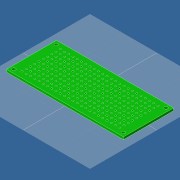
# Autodesk Inventor part: PCB_70x30
Saved by Autodesk Inventor 2016 SP2 (Build 200236200, 236)
## iProperties
Created: 2017-11-11
Part Number: PCB_70x30
Material: Generisch
Document SubType Name: Modeling
Designer: User
Density: 1 g/cm^3
Appearance: Dunkelgrün
Author: User
Autodesk Inventor part; units mm, degrees
ref_plane "YZ Plane" through (0, 0, 0) normal (1, 0, 0) x (0, 1, 0)
ref_plane "XZ Plane" through (0, 0, 0) normal (0, 1, 0) x (-1, 0, 0)
ref_plane "XY Plane" through (0, 0, 0) normal (0, 0, 1) x (1, 0, 0)
sketch "Skizze1" plane through (0, 0, 0) normal (0, 0, 1) x (1, 0, 0)
  line L0 (35, -15) -> (-35, -15)
  line L1 (-35, -15) -> (-35, 15)
  line L2 (-35, 15) -> (35, 15)
  line L3 (35, 15) -> (35, -15)
  line L4 (35, -15) -> (-35, 15) construction
  line L5 (-35, -15) -> (35, 15) construction
  circle A0 centre (-32.75, 12.75) radius 1
  circle A1 centre (-32.75, -12.75) radius 1
  circle A2 centre (32.75, 12.75) radius 1
  circle A3 centre (32.75, -12.75) radius 1
  line L6 (-49, 0) -> (49, 0) construction
  line L7 (0, -21) -> (0, 21) construction
  point P0 (0, 0)
  dimension "d0" = 70
  dimension "d1" = 30
  dimension "d45" = 2
  dimension "d46" = 65.5
  dimension "d47" = 25.5
  constraints: 12 end point, 4 centre point, 3 equal radius, 2 horizontal alignment, 2 midpoint, 2 parallel, 2 symmetric about line, 2 vertical alignment, 1 horizontal, 1 perpendicular
  measures "d0" distance of L1.end L2.end
  measures "d1" distance of L0.end L1.end
  measures "d45" diameter of A0
  measures "d46" distance of A2.centre A0.centre
  measures "d47" distance of A3.centre A2.centre
extrude "Extrusion1" add sketch "Skizze1" along normal blind 1.5 contours L0 L1 L2 L3 | A0 | A1 | A2 | A3
sketch "Skizze2" plane through (0, 0, 1.5) normal (0, 0, 1) x (1, 0, 0)
  line L0 (-49, 0) -> (49, 0) projected
  line L1 (0, -23.114) -> (0, 23.114) projected
  point P0 (0, 0)
  point P1 (-1.27, 1.27)
  point P2 (1.27, 1.27)
  point P3 (1.27, -1.27)
  point P4 (-1.27, -1.27)
  point P5 (-1.27, 3.81)
  point P6 (-1.27, 6.35)
  point P7 (-1.27, 8.89)
  point P8 (-1.27, 11.43)
  point P9 (-3.81, 1.27)
  point P10 (-3.81, 3.81)
  point P11 (-3.81, 6.35)
  point P12 (-3.81, 8.89)
  point P13 (-3.81, 11.43)
  point P14 (-6.35, 1.27)
  point P15 (-6.35, 3.81)
  point P16 (-6.35, 6.35)
  point P17 (-6.35, 8.89)
  point P18 (-6.35, 11.43)
  point P19 (-8.89, 1.27)
  point P20 (-8.89, 3.81)
  point P21 (-8.89, 6.35)
  point P22 (-8.89, 8.89)
  point P23 (-8.89, 11.43)
  point P24 (-11.43, 1.27)
  point P25 (-11.43, 3.81)
  point P26 (-11.43, 6.35)
  point P27 (-11.43, 8.89)
  point P28 (-11.43, 11.43)
  point P29 (-13.97, 1.27)
  point P30 (-13.97, 3.81)
  point P31 (-13.97, 6.35)
  point P32 (-13.97, 8.89)
  point P33 (-13.97, 11.43)
  point P34 (-16.51, 1.27)
  point P35 (-16.51, 3.81)
  point P36 (-16.51, 6.35)
  point P37 (-16.51, 8.89)
  point P38 (-16.51, 11.43)
  point P39 (-19.05, 1.27)
  point P40 (-19.05, 3.81)
  point P41 (-19.05, 6.35)
  point P42 (-19.05, 8.89)
  point P43 (-19.05, 11.43)
  point P44 (-21.59, 1.27)
  point P45 (-21.59, 3.81)
  point P46 (-21.59, 6.35)
  point P47 (-21.59, 8.89)
  point P48 (-21.59, 11.43)
  point P49 (-24.13, 1.27)
  point P50 (-24.13, 3.81)
  point P51 (-24.13, 6.35)
  point P52 (-24.13, 8.89)
  point P53 (-24.13, 11.43)
  point P54 (3.81, 1.27)
  point P55 (6.35, 1.27)
  point P56 (8.89, 1.27)
  point P57 (11.43, 1.27)
  point P58 (13.97, 1.27)
  point P59 (16.51, 1.27)
  point P60 (19.05, 1.27)
  point P61 (21.59, 1.27)
  point P62 (24.13, 1.27)
  point P63 (1.27, 3.81)
  point P64 (3.81, 3.81)
  point P65 (6.35, 3.81)
  point P66 (8.89, 3.81)
  point P67 (11.43, 3.81)
  point P68 (13.97, 3.81)
  point P69 (16.51, 3.81)
  point P70 (19.05, 3.81)
  point P71 (21.59, 3.81)
  point P72 (24.13, 3.81)
  point P73 (1.27, 6.35)
  point P74 (3.81, 6.35)
  point P75 (6.35, 6.35)
  point P76 (8.89, 6.35)
  point P77 (11.43, 6.35)
  point P78 (13.97, 6.35)
  point P79 (16.51, 6.35)
  point P80 (19.05, 6.35)
  point P81 (21.59, 6.35)
  point P82 (24.13, 6.35)
  point P83 (1.27, 8.89)
  point P84 (3.81, 8.89)
  point P85 (6.35, 8.89)
  point P86 (8.89, 8.89)
  point P87 (11.43, 8.89)
  point P88 (13.97, 8.89)
  point P89 (16.51, 8.89)
  point P90 (19.05, 8.89)
  point P91 (21.59, 8.89)
  point P92 (24.13, 8.89)
  point P93 (1.27, 11.43)
  point P94 (3.81, 11.43)
  point P95 (6.35, 11.43)
  point P96 (8.89, 11.43)
  point P97 (11.43, 11.43)
  point P98 (13.97, 11.43)
  point P99 (16.51, 11.43)
  point P100 (19.05, 11.43)
  point P101 (21.59, 11.43)
  point P102 (24.13, 11.43)
  point P103 (-1.27, -3.81)
  point P104 (-1.27, -6.35)
  point P105 (-1.27, -8.89)
  point P106 (-1.27, -11.43)
  point P107 (-3.81, -1.27)
  point P108 (-3.81, -3.81)
  point P109 (-3.81, -6.35)
  point P110 (-3.81, -8.89)
  point P111 (-3.81, -11.43)
  point P112 (-6.35, -1.27)
  point P113 (-6.35, -3.81)
  point P114 (-6.35, -6.35)
  point P115 (-6.35, -8.89)
  point P116 (-6.35, -11.43)
  point P117 (-8.89, -1.27)
  point P118 (-8.89, -3.81)
  point P119 (-8.89, -6.35)
  point P120 (-8.89, -8.89)
  point P121 (-8.89, -11.43)
  point P122 (-11.43, -1.27)
  point P123 (-11.43, -3.81)
  point P124 (-11.43, -6.35)
  point P125 (-11.43, -8.89)
  point P126 (-11.43, -11.43)
  point P127 (-13.97, -1.27)
  point P128 (-13.97, -3.81)
  point P129 (-13.97, -6.35)
  point P130 (-13.97, -8.89)
  point P131 (-13.97, -11.43)
  point P132 (-16.51, -1.27)
  point P133 (-16.51, -3.81)
  point P134 (-16.51, -6.35)
  point P135 (-16.51, -8.89)
  point P136 (-16.51, -11.43)
  point P137 (-19.05, -1.27)
  point P138 (-19.05, -3.81)
  point P139 (-19.05, -6.35)
  point P140 (-19.05, -8.89)
  point P141 (-19.05, -11.43)
  point P142 (-21.59, -1.27)
  point P143 (-21.59, -3.81)
  point P144 (-21.59, -6.35)
  point P145 (-21.59, -8.89)
  point P146 (-21.59, -11.43)
  point P147 (-24.13, -1.27)
  point P148 (-24.13, -3.81)
  point P149 (-24.13, -6.35)
  point P150 (-24.13, -8.89)
  point P151 (-24.13, -11.43)
  point P152 (1.27, -3.81)
  point P153 (1.27, -6.35)
  point P154 (1.27, -8.89)
  point P155 (1.27, -11.43)
  point P156 (3.81, -1.27)
  point P157 (3.81, -3.81)
  point P158 (3.81, -6.35)
  point P159 (3.81, -8.89)
  point P160 (3.81, -11.43)
  point P161 (6.35, -1.27)
  point P162 (6.35, -3.81)
  point P163 (6.35, -6.35)
  point P164 (6.35, -8.89)
  point P165 (6.35, -11.43)
  point P166 (8.89, -1.27)
  point P167 (8.89, -3.81)
  point P168 (8.89, -6.35)
  point P169 (8.89, -8.89)
  point P170 (8.89, -11.43)
  point P171 (11.43, -1.27)
  point P172 (11.43, -3.81)
  point P173 (11.43, -6.35)
  point P174 (11.43, -8.89)
  point P175 (11.43, -11.43)
  point P176 (13.97, -1.27)
  point P177 (13.97, -3.81)
  point P178 (13.97, -6.35)
  point P179 (13.97, -8.89)
  point P180 (13.97, -11.43)
  point P181 (16.51, -1.27)
  point P182 (16.51, -3.81)
  point P183 (16.51, -6.35)
  point P184 (16.51, -8.89)
  point P185 (16.51, -11.43)
  point P186 (19.05, -1.27)
  point P187 (19.05, -3.81)
  point P188 (19.05, -6.35)
  point P189 (19.05, -8.89)
  point P190 (19.05, -11.43)
  point P191 (21.59, -1.27)
  point P192 (21.59, -3.81)
  point P193 (21.59, -6.35)
  point P194 (21.59, -8.89)
  point P195 (21.59, -11.43)
  point P196 (24.13, -1.27)
  point P197 (24.13, -3.81)
  point P198 (24.13, -6.35)
  point P199 (24.13, -8.89)
  dimension "d4" = 2.54
  dimension "d5" = 2.54
  dimension "d8" = 2.54
  dimension "d11" = 2.54
  dimension "d16" = 2.54
  dimension "d19" = 2.54
  dimension "d24" = 2.54
  dimension "d27" = 2.54
  dimension "d32" = 2.54
  dimension "d35" = 2.54
  constraints: 4 horizontal, 4 vertical, 2 horizontal alignment, 2 symmetric about line, 2 vertical alignment, 236 other
  measures "d4" distance of point (1.27, 1.27) point (-1.27, 1.27)
  measures "d5" distance of point (-1.27, -1.27) point (-1.27, 1.27)
  measures "d8" distance of point (-1.27, 1.27) point (-1.27, 3.81)
  measures "d11" distance of point (-1.27, 1.27) point (-3.81, 1.27)
  measures "d16" distance of point (1.27, 1.27) point (3.81, 1.27)
  measures "d19" distance of point (1.27, 1.27) point (1.27, 3.81)
  measures "d24" distance of point (-1.27, -1.27) point (-1.27, -3.81)
  measures "d27" distance of point (-1.27, -1.27) point (-3.81, -1.27)
  measures "d32" distance of point (1.27, -1.27) point (1.27, -3.81)
  measures "d35" distance of point (1.27, -1.27) point (3.81, -1.27)
hole "Bohrung1" at (-1.27, 1.27, 1.5) at (1.27, 1.27, 1.5) at (1.27, -1.27, 1.5) at (-1.27, -1.27, 1.5) at (-1.27, 3.81, 1.5) at (-1.27, 6.35, 1.5) at (-1.27, 8.89, 1.5) at (-1.27, 11.43, 1.5) at (-3.81, 1.27, 1.5) at (-3.81, 3.81, 1.5) at (-3.81, 6.35, 1.5) at (-3.81, 8.89, 1.5) at (-3.81, 11.43, 1.5) at (-6.35, 1.27, 1.5) at (-6.35, 3.81, 1.5) at (-6.35, 6.35, 1.5) at (-6.35, 8.89, 1.5) at (-6.35, 11.43, 1.5) at (-8.89, 1.27, 1.5) at (-8.89, 3.81, 1.5) at (-8.89, 6.35, 1.5) at (-8.89, 8.89, 1.5) at (-8.89, 11.43, 1.5) at (-11.43, 1.27, 1.5) at (-11.43, 3.81, 1.5) at (-11.43, 6.35, 1.5) at (-11.43, 8.89, 1.5) at (-11.43, 11.43, 1.5) at (-13.97, 1.27, 1.5) at (-13.97, 3.81, 1.5) at (-13.97, 6.35, 1.5) at (-13.97, 8.89, 1.5) at (-13.97, 11.43, 1.5) at (-16.51, 1.27, 1.5) at (-16.51, 3.81, 1.5) at (-16.51, 6.35, 1.5) at (-16.51, 8.89, 1.5) at (-16.51, 11.43, 1.5) at (-19.05, 1.27, 1.5) at (-19.05, 3.81, 1.5) at (-19.05, 6.35, 1.5) at (-19.05, 8.89, 1.5) at (-19.05, 11.43, 1.5) at (-21.59, 1.27, 1.5) at (-21.59, 3.81, 1.5) at (-21.59, 6.35, 1.5) at (-21.59, 8.89, 1.5) at (-21.59, 11.43, 1.5) at (-24.13, 1.27, 1.5) at (-24.13, 3.81, 1.5) direction (0, 0, -1) diameter 1 end through all and at (-24.13, 6.35, 1.5) (-24.13, 8.89, 1.5) (-24.13, 11.43, 1.5) (3.81, 1.27, 1.5) (6.35, 1.27, 1.5) (8.89, 1.27, 1.5) (11.43, 1.27, 1.5) (13.97, 1.27, 1.5) (16.51, 1.27, 1.5) (19.05, 1.27, 1.5) (21.59, 1.27, 1.5) (24.13, 1.27, 1.5) (1.27, 3.81, 1.5) (3.81, 3.81, 1.5) (6.35, 3.81, 1.5) (8.89, 3.81, 1.5) (11.43, 3.81, 1.5) (13.97, 3.81, 1.5) (16.51, 3.81, 1.5) (19.05, 3.81, 1.5) (21.59, 3.81, 1.5) (24.13, 3.81, 1.5) (1.27, 6.35, 1.5) (3.81, 6.35, 1.5) (6.35, 6.35, 1.5) (8.89, 6.35, 1.5) (11.43, 6.35, 1.5) (13.97, 6.35, 1.5) (16.51, 6.35, 1.5) (19.05, 6.35, 1.5) (21.59, 6.35, 1.5) (24.13, 6.35, 1.5) (1.27, 8.89, 1.5) (3.81, 8.89, 1.5) (6.35, 8.89, 1.5) (8.89, 8.89, 1.5) (11.43, 8.89, 1.5) (13.97, 8.89, 1.5) (16.51, 8.89, 1.5) (19.05, 8.89, 1.5) (21.59, 8.89, 1.5) (24.13, 8.89, 1.5) (1.27, 11.43, 1.5) (3.81, 11.43, 1.5) (6.35, 11.43, 1.5) (8.89, 11.43, 1.5) (11.43, 11.43, 1.5) (13.97, 11.43, 1.5) (16.51, 11.43, 1.5) (19.05, 11.43, 1.5) (21.59, 11.43, 1.5) (24.13, 11.43, 1.5) (-1.27, -3.81, 1.5) (-1.27, -6.35, 1.5) (-1.27, -8.89, 1.5) (-1.27, -11.43, 1.5) (-3.81, -1.27, 1.5) (-3.81, -3.81, 1.5) (-3.81, -6.35, 1.5) (-3.81, -8.89, 1.5) (-3.81, -11.43, 1.5) (-6.35, -1.27, 1.5) (-6.35, -3.81, 1.5) (-6.35, -6.35, 1.5) (-6.35, -8.89, 1.5) (-6.35, -11.43, 1.5) (-8.89, -1.27, 1.5) (-8.89, -3.81, 1.5) (-8.89, -6.35, 1.5) (-8.89, -8.89, 1.5) (-8.89, -11.43, 1.5) (-11.43, -1.27, 1.5) (-11.43, -3.81, 1.5) (-11.43, -6.35, 1.5) (-11.43, -8.89, 1.5) (-11.43, -11.43, 1.5) (-13.97, -1.27, 1.5) (-13.97, -3.81, 1.5) (-13.97, -6.35, 1.5) (-13.97, -8.89, 1.5) (-13.97, -11.43, 1.5) (-16.51, -1.27, 1.5) (-16.51, -3.81, 1.5) (-16.51, -6.35, 1.5) (-16.51, -8.89, 1.5) (-16.51, -11.43, 1.5) (-19.05, -1.27, 1.5) (-19.05, -3.81, 1.5) (-19.05, -6.35, 1.5) (-19.05, -8.89, 1.5) (-19.05, -11.43, 1.5) (-21.59, -1.27, 1.5) (-21.59, -3.81, 1.5) (-21.59, -6.35, 1.5) (-21.59, -8.89, 1.5) (-21.59, -11.43, 1.5) (-24.13, -1.27, 1.5) (-24.13, -3.81, 1.5) (-24.13, -6.35, 1.5) (-24.13, -8.89, 1.5) (-24.13, -11.43, 1.5) (1.27, -3.81, 1.5) (1.27, -6.35, 1.5) (1.27, -8.89, 1.5) (1.27, -11.43, 1.5) (3.81, -1.27, 1.5) (3.81, -3.81, 1.5) (3.81, -6.35, 1.5) (3.81, -8.89, 1.5) (3.81, -11.43, 1.5) (6.35, -1.27, 1.5) (6.35, -3.81, 1.5) (6.35, -6.35, 1.5) (6.35, -8.89, 1.5) (6.35, -11.43, 1.5) (8.89, -1.27, 1.5) (8.89, -3.81, 1.5) (8.89, -6.35, 1.5) (8.89, -8.89, 1.5) (8.89, -11.43, 1.5) (11.43, -1.27, 1.5) (11.43, -3.81, 1.5) (11.43, -6.35, 1.5) (11.43, -8.89, 1.5) (11.43, -11.43, 1.5) (13.97, -1.27, 1.5) (13.97, -3.81, 1.5) (13.97, -6.35, 1.5) (13.97, -8.89, 1.5) (13.97, -11.43, 1.5) (16.51, -1.27, 1.5) (16.51, -3.81, 1.5) (16.51, -6.35, 1.5) (16.51, -8.89, 1.5) (16.51, -11.43, 1.5) (19.05, -1.27, 1.5) (19.05, -3.81, 1.5) (19.05, -6.35, 1.5) (19.05, -8.89, 1.5) (19.05, -11.43, 1.5) (21.59, -1.27, 1.5) (21.59, -3.81, 1.5) (21.59, -6.35, 1.5) (21.59, -8.89, 1.5) (21.59, -11.43, 1.5) (24.13, -1.27, 1.5) (24.13, -3.81, 1.5) (24.13, -6.35, 1.5) (24.13, -8.89, 1.5) (24.13, -11.43, 1.5) (-26.67, -11.43, 1.5) (-29.21, -11.43, 1.5) (-29.21, -8.89, 1.5) (-26.67, -8.89, 1.5) (-26.67, -6.35, 1.5) (-29.21, -6.35, 1.5) (-29.21, -3.81, 1.5) (-26.67, -3.81, 1.5) (-26.67, -1.27, 1.5) (-29.21, -1.27, 1.5) (-29.21, 11.43, 1.5) (-26.67, 11.43, 1.5) (-29.21, 8.89, 1.5) (-29.21, 6.35, 1.5) (-29.21, 3.81, 1.5) (-29.21, 1.27, 1.5) (-26.67, 3.81, 1.5) (-26.67, 6.35, 1.5) (-26.67, 8.89, 1.5) (26.67, 11.43, 1.5) (29.21, 11.43, 1.5) (29.21, 8.89, 1.5) (26.67, 8.89, 1.5) (26.67, 6.35, 1.5) (29.21, 6.35, 1.5) (29.21, -11.43, 1.5) (26.67, -11.43, 1.5) (26.67, -8.89, 1.5) (26.67, -6.35, 1.5) (29.21, -6.35, 1.5) (29.21, -8.89, 1.5) (26.67, -3.81, 1.5) (29.21, -3.81, 1.5) (26.67, -1.27, 1.5) (29.21, -1.27, 1.5) (26.67, 1.27, 1.5) (26.67, 3.81, 1.5) (29.21, 3.81, 1.5) (29.21, 1.27, 1.5) (-26.67, 1.27, 1.5)
extrude "Extrusion2" cut sketch "Skizze1" along normal through all contours A0 | A1 | A2 | A3
